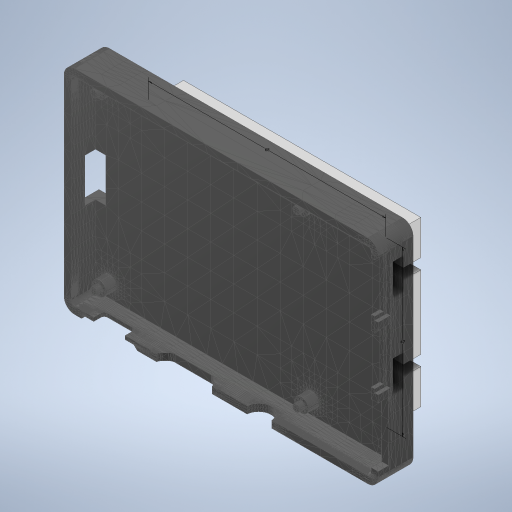
# Autodesk Inventor part: Inferior
Saved by Autodesk Inventor 2023 (Build 270158000, 158)
## iProperties
Created: 2022-06-21
Part Number: Inferior
Material: Generic
Document SubType Name: Modeling
Designer: nikol
Density: 1 g/cm^3
Appearance: Default
Author: nikol
Autodesk Inventor part; units mm, degrees
ref_plane "YZ Plane" through (0, 0, 0) normal (1, 0, 0) x (0, 1, 0)
ref_plane "XZ Plane" through (0, 0, 0) normal (0, 1, 0) x (-1, 0, 0)
ref_plane "XY Plane" through (0, 0, 0) normal (0, 0, 1) x (1, 0, 0)
sketch "Sketch1" plane through (-41, -6, 0) normal (0, 0, -1) x (-1, 0, 0)
  line L0 (-10.2196, -17.8058) -> (-78.2196, -17.8058)
  line L1 (-78.2196, -17.8058) -> (-78.2196, 29.1942)
  line L2 (-78.2196, 29.1942) -> (-10.2196, 29.1942)
  line L3 (-10.2196, 29.1942) -> (-10.2196, -17.8058)
  point P0 (-41, 6)
  dimension "d0" = 68
  dimension "d1" = 47
  constraints: 8 end point, 2 parallel, 1 horizontal, 1 perpendicular
  measures "d0" distance of L1.end L2.end
  measures "d1" distance of L0.end L1.end
extrude "Extrusion1" add sketch "Sketch1" along normal blind 10
sketch "Sketch2" plane through (37.2196, -23.8058, 0) normal (1, 0, 0) x (0, 0, -1)
  line L0 (0, 47) -> (10, 47) projected
  line L1 (10, 47) -> (10, 37) construction
  line L2 (10, 47) -> (10, 0) projected
  line L3 (10, 37) -> (5, 37)
  line L4 (5, 37) -> (5, 40)
  line L5 (5, 40) -> (2, 40)
  line L6 (10, 37) -> (10, 34)
  line L7 (10, 34) -> (5, 34)
  line L8 (5, 34) -> (5, 31)
  line L9 (5, 31) -> (2, 31)
  line L10 (2, 31) -> (2, 37)
  line L11 (0, 0) -> (10, 0) projected
  line L12 (10, 0) -> (10, 10) construction
  line L13 (10, 10) -> (5, 10)
  line L14 (5, 10) -> (5, 7)
  line L15 (5, 7) -> (2, 7)
  line L16 (2, 7) -> (2, 16)
  line L17 (2, 16) -> (5, 16)
  line L18 (5, 16) -> (5, 13)
  line L19 (5, 13) -> (10, 13)
  line L20 (10, 13) -> (10, 10)
  line L21 (10, 13) -> (5, 13)
  line L22 (10, 37) -> (10, 34)
  point P0 (0, 23.8058)
  dimension "d4" = 10
  dimension "d6" = 3
  dimension "d7" = 3
  dimension "d8" = 3
  dimension "d9" = 3
  dimension "d10" = 6
  dimension "d11" = 10
  dimension "d12" = 5
  dimension "d13" = 3
  dimension "d14" = 3
  dimension "d15" = 9
  dimension "d16" = 3
  dimension "d17" = 3
  dimension "d18" = 5
  constraints: 40 end point, 8 perpendicular, 6 point on line, 3 horizontal, 2 collinear, 1 vertical
  measures "d4" distance of L0.end L1.end
  measures "d6" distance of L3.end L4.end
  measures "d7" distance of L4.end L5.end
  measures "d8" distance of L1.end L6.end
  measures "d9" distance of L7.end L8.end
  measures "d10" distance of L9.end L10.end
  measures "d11" distance of L2.end L12.end
  measures "d12" distance of L12.end L13.end
  measures "d13" distance of L13.end L14.end
  measures "d14" distance of L14.end L15.end
  measures "d15" distance of L15.end L16.end
  measures "d16" distance of L16.end L17.end
  measures "d17" distance of L17.end L18.end
  measures "d18" distance of L18.end L19.end
extrude "Extrusion2" cut sketch "Sketch2" against normal blind 68
sketch "Sketch3" plane through (37.2196, -23.8058, 0) normal (1, 0, 0) x (0, 0, -1)
  point P0 (0, 23.8058)
sketch "Sketch4" plane through (37.2196, -23.8058, 0) normal (1, 0, 0) x (0, 0, -1)
  line L0 (0, 47) -> (10, 47) projected
  line L1 (10, 47) -> (10, 37) construction
  line L2 (10, 47) -> (10, 13) projected
  line L3 (10, 37) -> (5, 37)
  line L4 (5, 37) -> (5, 40)
  line L5 (5, 40) -> (2, 40)
  line L6 (2, 40) -> (2, 31)
  line L7 (2, 31) -> (5, 31)
  line L8 (5, 31) -> (5, 34)
  line L9 (5, 34) -> (10, 34)
  line L10 (10, 37) -> (10, 34)
  point P0 (0, 23.8058)
  dimension "d21" = 10
  dimension "d22" = 5
  dimension "d23" = 3
  dimension "d24" = 3
  dimension "d25" = 9
  dimension "d26" = 3
  dimension "d27" = 3
  constraints: 18 end point, 4 point on line, 3 perpendicular, 1 collinear, 1 horizontal, 1 parallel
  measures "d21" distance of L0.end L1.end
  measures "d22" distance of L1.end L3.end
  measures "d23" distance of L3.end L4.end
  measures "d24" distance of L4.end L5.end
  measures "d25" distance of L5.end L6.end
  measures "d26" distance of L6.end L7.end
  measures "d27" distance of L7.end L8.end
extrude "Extrusion3" cut sketch "Sketch4" against normal blind 68
body "Solid1"
